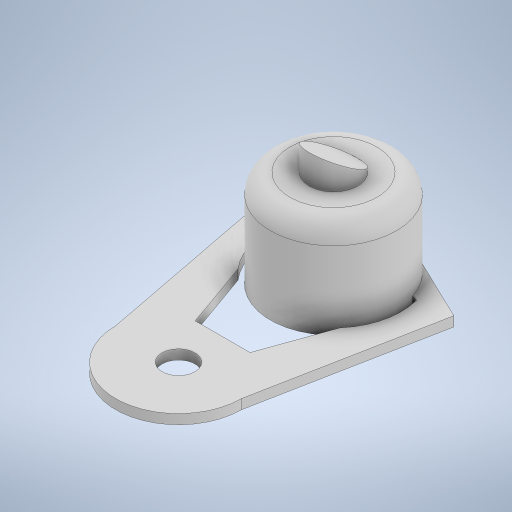
# Autodesk Inventor part: Sicherheitsgitter_Feder
Saved by Autodesk Inventor 2023 (Build 270158000, 158)
## iProperties
Created: 2023-03-30
Part Number: Sicherheitsgitter_Feder
Material: Generisch
Document SubType Name: Modeling
Designer: prigge
Density: 1 g/cm^3
Appearance: Vorgabe
Author: prigge
Autodesk Inventor part; units mm, degrees
ref_plane "YZ Plane" through (0, 0, 0) normal (1, 0, 0) x (0, 1, 0)
ref_plane "XZ Plane" through (0, 0, 0) normal (0, 1, 0) x (-1, 0, 0)
ref_plane "XY Plane" through (0, 0, 0) normal (0, 0, 1) x (1, 0, 0)
sketch "Skizze1" plane through (0, 0, 0) normal (0, 1, 0) x (-1, 0, 0)
  circle A0 centre (0, 0) radius 1.7
  arc A1 (6.5, 0) -> (-6.5, 0) centre (0, 0) ccw
  line L0 (6.5, 0) -> (6.5, -16)
  arc A2 (-6.5, -16) -> (6.5, -16) centre (0, -16) ccw
  line L1 (-6.5, -16) -> (-6.5, 0)
  dimension "d0" = 13
  dimension "d1" = 3.4
  dimension "d2" = 16
  constraints: 5 point on circle, 4 end point, 4 tangent, 3 centre point, 2 coincident, 2 vertical
  measures "d0" distance between parallel lines of L1 L0
  measures "d1" diameter of A0
  measures "d2" distance of A2.centre point (0, 0)
extrude "Extrusion1" add sketch "Skizze1" along normal blind 1
sketch "Skizze2" plane through (0, 1, 0) normal (0, 1, 0) x (1, 0, 0)
  arc A0 (6.5, 16) -> (-6.5, 16) centre (0, 16) ccw projected
  circle A1 centre (0, 16) radius 6.5
  point P0 (0, 0)
  point P1 (6.5, 16)
  constraints: 1 centre point, 1 coincident
extrude "Extrusion2" add sketch "Skizze2" along normal blind 9
sketch "Skizze3" plane through (0, 10, -16) normal (0, 1, 0) x (1, 0, 0)
  circle A0 centre (0, 0) radius 2.5
  point P0 (0, -16)
  dimension "d7" = 5
  constraints: 1 centre point
  measures "d7" diameter of A0
extrude "Extrusion3" add sketch "Skizze3" along normal blind 3
sketch "Skizze4" plane through (0, 0, 0) normal (1, 0, 0) x (0, 1, 0)
  line L0 (1, 6.5) -> (1, 1.7) projected
  line L1 (1, 1.7) -> (0, 1.7) projected
  line L2 (0, 1.7) -> (0, 6.5) projected
  line L3 (0, 6.5) -> (1, 6.5) projected
  line L4 (1, -1.7) -> (1, -9.5) projected
  line L5 (1, -9.5) -> (10, -9.5) projected
  line L6 (10, -9.5) -> (10, -13.5) projected
  line L7 (10, -13.5) -> (13, -13.5) projected
  line L8 (13, -13.5) -> (13, -18.5) projected
  line L9 (13, -18.5) -> (10, -18.5) projected
  line L10 (10, -18.5) -> (10, -22.5) projected
  line L11 (10, -22.5) -> (0, -22.5) projected
  line L12 (0, -22.5) -> (0, -1.7) projected
  line L13 (0, -1.7) -> (1, -1.7) projected
  line L14 (13, -18.5) -> (13, -13.5) projected
  line L15 (10, -18.5) -> (13, -13.5)
  point P0 (0, 0)
  constraints: 2 end point
extrude "Extrusion4" cut sketch "Skizze4" along normal through all both and the other way through all contours L8 L9 L15
fillet "Rundung1" radius 2 3 edges at (-1.2748, 10, -9.6262) (6.3738, 10, -17.2748) (0, 10, -22.5)
sketch "Skizze6" plane through (0, 0, 0) normal (0, 1, 0) x (-1, 0, 0)
  line L0 (6.5, -16) -> (6.5, 0) projected
  line L1 (6.5, 0) -> (10.0547, -18.3705)
  line L2 (10.0547, -18.3705) -> (2.8215, -21.8557)
  arc A0 (-6.5, -16) -> (6.5, -16) centre (0, -16) ccw projected
  point P0 (0, 0)
  constraints: 4 end point, 1 point on circle, 1 tangent
extrude "Extrusion6" add sketch "Skizze6" along normal up to surface (1 mm away)
mirror "Spiegeln2" about plane through (0, 0, 0) normal (1, 0, 0) of "Extrusion6"
sketch "Skizze7" plane through (0, 0, 0) normal (0, 1, 0) x (-1, 0, 0)
  circle A0 centre (0, -16) radius 6.5 projected
  arc A1 (2.8215, -21.8557) -> (-2.8215, -21.8557) centre (0, -16) ccw projected
  line L0 (2.8333, -4.5583) -> (0, -4.5583)
  line L1 (0, -4.5583) -> (0, -9.5)
  arc A2 (6.749, -17.8097) -> (5.214, -11.3483) centre (0, -16) ccw
  line L2 (5.2667, -11.408) -> (2.8333, -4.5583)
  line L3 (6.749, -17.8097) -> (6.1809, -18.0115)
  point P0 (0, 0)
  constraints: 8 end point, 5 point on circle, 1 centre point, 1 coincident, 1 horizontal, 1 perpendicular, 1 tangent
extrude "Extrusion7" cut sketch "Skizze7" along normal blind 10 contours A0 L1 L0 L2 A2 L3
mirror "Spiegeln3" about plane through (0, 0, 0) normal (1, 0, 0) of "Extrusion7"
